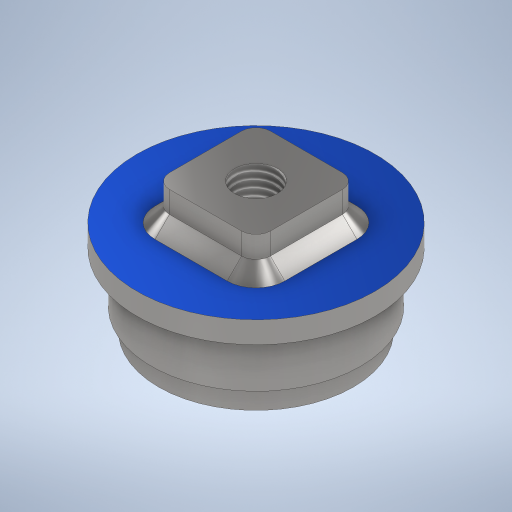
# Autodesk Inventor part: Top_contact
Saved by Autodesk Inventor 2023 (Build 270158000, 158)
## iProperties
Created: 2022-09-21
Part Number: Top_contact
Material: Сталь нержавеющая AISI 202
Document SubType Name: Modeling
Designer: Makar
Density: 7.85472 g/cm^3
Appearance: С умеренной полировкой
Mass: 74.4204 g
Surface Area: 34.0302 cm^2
Volume: 9.4746 cm^3
Author: Makar
Autodesk Inventor part; units mm, degrees
ref_plane "YZ Plane" through (0, 0, 0) normal (1, 0, 0) x (0, 1, 0)
ref_plane "XZ Plane" through (0, 0, 0) normal (0, 1, 0) x (-1, 0, 0)
ref_plane "XY Plane" through (0, 0, 0) normal (0, 0, 1) x (1, 0, 0)
sketch "Эскиз1" plane through (0, 0, 0) normal (0, 0, 1) x (1, 0, 0)
  line L0 (0, 0) -> (0, 13)
  line L1 (0, 13) -> (16.5, 13)
  line L2 (16.5, 13) -> (16.5, 10)
  line L3 (16.5, 10) -> (14.5, 10)
  line L4 (14.5, 10) -> (14.5, 3)
  line L5 (14.5, 3) -> (13.5, 3)
  line L6 (13.5, 3) -> (13.5, 0)
  line L7 (13.5, 0) -> (0, 0)
  dimension "d0" = 13
  dimension "d1" = 16.5
  dimension "d2" = 3
  dimension "d3" = 2
  dimension "d4" = 7
  dimension "d5" = 1
  constraints: 16 end point, 7 perpendicular, 1 vertical
  measures "d0" distance of L0.start L0.end
  measures "d1" distance of L0.end L1.end
  measures "d2" distance of L1.end L2.end
  measures "d3" distance of L2.end L3.end
  measures "d4" distance of L3.end L4.end
  measures "d5" distance of L4.end L5.end
revolve "Вращение1" add sketch "Эскиз1" angle 360 about axis through (0, 0, 0) along (0, 1, 0)
sketch "Эскиз2" plane through (0, 13, 0) normal (0, 1, 0) x (1, 0, 0)
  circle A0 centre (0, 0) radius 3
  line L0 (-5, -7) -> (5, -7)
  line L1 (7, -5) -> (7, 5)
  line L2 (5, 7) -> (-5, 7)
  line L3 (-7, 5) -> (-7, -5)
  line L4 (-7, -7) -> (7, 7) construction
  line L5 (7, -7) -> (-7, 7) construction
  arc A1 (-7, -5) -> (-5, -7) centre (-5, -5) ccw
  arc A2 (5, -7) -> (7, -5) centre (5, -5) ccw
  arc A3 (7, 5) -> (5, 7) centre (5, 5) ccw
  arc A4 (-5, 7) -> (-7, 5) centre (-5, 5) ccw
  dimension "d7" = 6
  dimension "d8" = 14
  dimension "d9" = 14
  dimension "d10" = 2
  constraints: 12 end point, 8 point on circle, 8 point on line, 8 tangent, 5 centre point, 3 equal radius, 2 midpoint, 2 parallel, 1 coincident, 1 horizontal, 1 perpendicular
  measures "d7" diameter of A0
  measures "d8" distance of L5.end L4.end
  measures "d9" distance of L4.end L5.start
  measures "d10" radius of A1
extrude "Выдавливание1" cut sketch "Эскиз2" against normal blind 24 contours A0
extrude "Выдавливание2" add sketch "Эскиз2" along normal blind 5
chamfer "Фаска1" distance 2 angle 45 8 edges at (0, 13, 7) (-6.4142, 13, 6.4142) (-7, 13, 0) (-6.4142, 13, -6.4142) (0, 13, -7) (6.4142, 13, -6.4142) (7, 13, 0) (6.4142, 13, 6.4142)
thread "Резьба1" size "M6x1" class "6H" standard "ANSI Metric M Profile" full length
